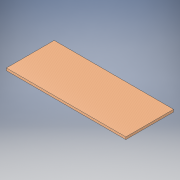
# Autodesk Inventor part: Part6
Saved by Autodesk Inventor 2019 (Build 230136000, 136)
## iProperties
Created: 2022-01-28
Part Number: Part6
Material: Generic
Document SubType Name: Modeling
Designer: Sepehr
Density: 1 g/cm^3
Appearance: Default
Author: Sepehr
Autodesk Inventor part; units mm, degrees
ref_plane "YZ Plane" through (0, 0, 0) normal (1, 0, 0) x (0, 1, 0)
ref_plane "XZ Plane" through (0, 0, 0) normal (0, 1, 0) x (-1, 0, 0)
ref_plane "XY Plane" through (0, 0, 0) normal (0, 0, 1) x (1, 0, 0)
sketch "Sketch1" plane through (0, 0, 0) normal (0, 1, 0) x (-1, 0, 0)
  line L0 (-12500, -5000) -> (12500, -5000)
  line L1 (12500, -5000) -> (12500, 5000)
  line L2 (12500, 5000) -> (-12500, 5000)
  line L3 (-12500, 5000) -> (-12500, -5000)
  line L4 (-12500, -5000) -> (12500, 5000) construction
  line L5 (12500, -5000) -> (-12500, 5000) construction
  point P0 (0, 0)
  dimension "d0" = 25000
  dimension "d1" = 10000
  constraints: 12 end point, 2 midpoint, 2 parallel, 1 horizontal, 1 perpendicular
  measures "d0" distance of L2.end L1.end
  measures "d1" distance of L1.end L0.end
extrude "Extrusion1" add sketch "Sketch1" along normal blind 500
body "Solid1"
